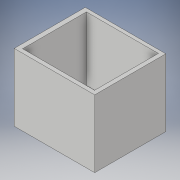
# Autodesk Inventor part: tray2
Saved by Autodesk Inventor 2019 (Build 230136000, 136)
## iProperties
Created: 2020-02-19
Part Number: tray2
Material: Generic
Document SubType Name: Modeling
Designer: Dell
Density: 1 g/cm^3
Appearance: Default
Author: Dell
Autodesk Inventor part; units mm, degrees
ref_plane "YZ Plane" through (0, 0, 0) normal (1, 0, 0) x (0, 1, 0)
ref_plane "XZ Plane" through (0, 0, 0) normal (0, 1, 0) x (-1, 0, 0)
ref_plane "XY Plane" through (0, 0, 0) normal (0, 0, 1) x (1, 0, 0)
sketch "Sketch1" plane through (0, 0, 0) normal (0, 1, 0) x (-1, 0, 0)
  line L0 (-81.4912, -78.8023) -> (133.5088, -78.8023)
  line L1 (133.5088, -78.8023) -> (133.5088, 111.1977)
  line L2 (133.5088, 111.1977) -> (-81.4912, 111.1977)
  line L3 (-81.4912, 111.1977) -> (-81.4912, -78.8023)
  point P0 (0, 0)
  dimension "d0" = 190
  dimension "d1" = 215
  constraints: 8 end point, 2 parallel, 1 horizontal, 1 perpendicular
  measures "d0" distance of L2.end L0.start
  measures "d1" distance of L0.start L0.end
extrude "Extrusion1" add sketch "Sketch1" along normal blind 180
sketch "Sketch2" plane through (0, 180, 0) normal (0, 1, 0) x (1, 0, 0)
  line L0 (70.7245, -100.7611) -> (-121.4246, -100.7611)
  line L1 (-121.4246, -100.7611) -> (-121.4246, 69.6594)
  line L2 (-121.4246, 69.6594) -> (70.7245, 69.6594)
  line L3 (70.7245, 69.6594) -> (70.7245, -100.7611)
  point P0 (0, 0)
  constraints: 8 end point, 2 parallel, 1 horizontal, 1 perpendicular
extrude "Extrusion2" cut sketch "Sketch2" along normal mid plane 340
body "Solid1"
